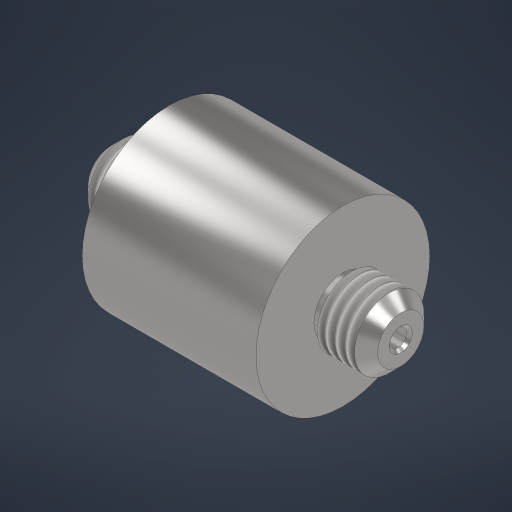
# Autodesk Inventor part: HM1-1002
Saved by Autodesk Inventor 2024.3 (Build 283343000, 343)
## iProperties
Created: 2023-12-03
Part Number: HM1-1002
Material: Steel, Alloy
Document SubType Name: Modeling
Designer: fablabadmin
Density: 7.73 g/cm^3
Appearance: Semi-Polished
Description: Head
Author: fablabadmin
Autodesk Inventor part; units mm, degrees
ref_plane "YZ Plane" through (0, 0, 0) normal (1, 0, 0) x (0, 1, 0)
ref_plane "XZ Plane" through (0, 0, 0) normal (0, 1, 0) x (-1, 0, 0)
ref_plane "XY Plane" through (0, 0, 0) normal (0, 0, 1) x (1, 0, 0)
sketch "Sketch1" plane through (0, 0, 0) normal (0, 0, 1) x (1, 0, 0)
  line L0 (-35, 0) -> (35, 0) construction
  line L1 (0, -21) -> (0, 21) construction
  line L2 (0, 15) -> (-15, 15)
  line L3 (-15, 15) -> (-15, 5)
  line L4 (-15, 5) -> (-16, 5)
  line L5 (-16, 5) -> (-16.5774, 6)
  line L6 (-16.5774, 6) -> (-25, 6)
  line L7 (-25, 6) -> (-25, 0)
  line L8 (0, 15) -> (15, 15)
  line L9 (15, 15) -> (15, 5)
  line L10 (15, 5) -> (16, 5)
  line L11 (16, 5) -> (16.5774, 6)
  line L12 (16.5774, 6) -> (25, 6)
  line L13 (25, 6) -> (25, 0)
  line L14 (0, -15) -> (-15, -15)
  line L15 (-15, -15) -> (-15, -5)
  line L16 (-15, -5) -> (-16, -5)
  line L17 (-16, -5) -> (-16.5774, -6)
  line L18 (-16.5774, -6) -> (-25, -6)
  line L19 (-25, -6) -> (-25, 0)
  line L20 (15, -15) -> (15, -5)
  line L21 (15, -5) -> (16, -5)
  line L22 (16, -5) -> (16.5774, -6)
  line L23 (16.5774, -6) -> (25, -6)
  line L24 (25, -6) -> (25, 0)
  line L25 (0, -15) -> (15, -15)
  line L26 (-9, -15) -> (-9, -11)
  line L27 (-9, -11) -> (-5, -11)
  line L28 (-5, -11) -> (-5, 8)
  line L29 (-5, 8) -> (0, 11.0043)
  line L30 (0, 11.0043) -> (0, -15)
  line L31 (-25, 0) -> (25, 0)
  line L32 (-25, 1.5) -> (25, 1.5)
  point P0 (0, 0)
  dimension "d0" = 30
  dimension "d1" = 12
  dimension "d3" = 8.4227
  dimension "d5" = 60
  dimension "d6" = 10
  dimension "d7" = 30
  dimension "d8" = 50
  dimension "d9" = 59
  dimension "d10" = 10
  dimension "d11" = 4
  dimension "d12" = 18
  dimension "d13" = 23
  dimension "d23" = 3
  dimension "d27" = 10
  dimension "d29" = 1
  constraints: 62 end point, 17 symmetric about line, 7 perpendicular, 6 point on line, 1 collinear, 1 horizontal, 1 parallel, 1 vertical
  measures "d0" diameter of L2 L0
  measures "d1" diameter of L6 L0
  measures "d3" distance from line of L5.end L7
  measures "d5" angle of L4 L5
  measures "d6" diameter of L4 L0
  measures "d7" diameter of L3 L1
  measures "d8" diameter of L7 L1
  measures "d9" angle of L1 L29
  measures "d10" diameter of L28 L1
  measures "d11" distance of L26.start L26.end
  measures "d12" diameter of L26 L1
  measures "d13" distance from line of L14 L28.end
  measures "d23" diameter of L32 L0
  measures "d27" distance between parallel lines of L3 L7
  measures "d29" distance from line of L4.end L3
revolve "Revolution1" add sketch "Sketch1" angle 360 about axis through (-25, 0, 0) along (1, 0, 0) contours L8 L9 L10 L11 L12 L13 L32 L30 L29 L28 L7 L6 L5 L4 L3 L2 | L28 L29 L30 L32
revolve "Revolution2" cut sketch "Sketch1" angle 360 about axis through (0, 11.0043, 0) along (0, -1, 0) contours L32 L30 L31 L28 | L28 L29 L30 L32 | L31 L30 L14 L26 L27 L28
thread "Thread2" size "M12x1.75" class "6g" standard "ISO Metric profile" full length
chamfer "Chamfer1" distance 2 angle 45 2 edges at (-25, -6, 0) (25, -6, 0)
chamfer "Chamfer2" distance 0.5 angle 45 2 edges at (-25, -1.5, 0) (25, -1.5, 0)
sketch "Sketch2" plane through (0, -11, 0) normal (0, -1, 0) x (0, 0, -1)
  circle A0 centre (0, 0) radius 5 projected
  point P0 (0, 0)
  constraints: 1 coincident
hole "Hole1" at (0, -11, 0) direction (0, 1, 0) diameter 10.106 depth 20 tip angle 118 countersink diameter 13 countersink angle 90 thread size "M12x1.75" class "6H" standard "ISO Metric profile"
body "Solid1"
